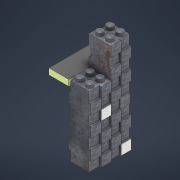
# Autodesk Inventor part: 110033226_ipt_34_中心城堡圍牆
Saved by Autodesk Inventor 2022 (Build 260153000, 153)
## iProperties
Created: 2022-06-24
Part Number: 110033226_ipt_34_中心城堡圍牆
Material: 一般
Document SubType Name: Modeling
Designer: User
Density: 1 g/cm^3
Appearance: 預設
Author: User
Autodesk Inventor part; units mm, degrees
ref_plane "YZ Plane" through (0, 0, 0) normal (1, 0, 0) x (0, 1, 0)
ref_plane "XZ Plane" through (0, 0, 0) normal (0, 1, 0) x (-1, 0, 0)
ref_plane "XY Plane" through (0, 0, 0) normal (0, 0, 1) x (1, 0, 0)
sketch "草圖1" plane through (0, 0, 0) normal (0, 1, 0) x (-1, 0, 0)
  line L0 (2.5, 10) -> (-2.5, 10)
  line L1 (-2.5, 10) -> (-2.5, -10)
  line L2 (-2.5, -10) -> (2.5, -10)
  line L3 (2.5, -10) -> (2.5, 10)
  circle A0 centre (0, 7.5) radius 1.7
  circle A1 centre (0, 2.5) radius 1.7
  circle A2 centre (0, -2.5) radius 1.7
  circle A3 centre (0, -7.5) radius 1.7
  line L4 (2.5, 0) -> (-2.5, 0)
  point P0 (0, 0)
  point P1 (0, -10)
  dimension "d0" = 5
  dimension "d1" = 20
  dimension "d2" = 3.4
  dimension "d3" = 2.5
  dimension "d4" = 2.5
  dimension "d7" = 5
  constraints: 10 end point, 4 centre point, 3 midpoint, 2 parallel, 1 horizontal, 1 horizontal alignment, 1 perpendicular, 1 vertical, 1 vertical alignment, 6 other
  measures "d0" distance of L2.end L1.end
  measures "d1" distance of L1.end L0.end
  measures "d2" diameter of A0
  measures "d3" distance from line of L3 A0.centre
  measures "d4" distance from line of L0 A0.centre
  measures "d7" distance of A0.centre A1.centre
extrude "擠出1" add sketch "草圖1" along normal blind 35 contours L3 L4 L1 L0 | A0 | A1
extrude "擠出2" cut sketch "草圖1" along normal blind 1.5 contours A0 | A1
extrude "擠出3" add sketch "草圖1" along normal blind 50 contours L3 L2 L1 L4 | A2 | A3
extrude "擠出4" cut sketch "草圖1" along normal blind 1.5 contours A2 | A3
sketch "草圖2" plane through (0, 50, 0) normal (0, 1, 0) x (1, 0, 0)
  circle A0 centre (0, 7.5) radius 1.7 projected
  circle A1 centre (0, 2.5) radius 1.7 projected
  point P0 (0, 0)
extrude "擠出5" add sketch "草圖2" along normal blind 1.5
sketch "草圖3" plane through (0, 35, 0) normal (0, 1, 0) x (1, 0, 0)
  circle A0 centre (0, -2.5) radius 1.7 projected
  circle A1 centre (0, -7.5) radius 1.7 projected
  point P0 (0, 0)
extrude "擠出6" add sketch "草圖3" along normal blind 1.5
pattern_linear "矩形陣列1" count 2 spacing 5 along (1, 0, 0) of "擠出6", "擠出5", "擠出4", "擠出3", "擠出2", "擠出1"
sketch "草圖5" plane through (7.5, 0, 10) normal (1, 0, 0) x (0, 0, -1)
  line L0 (0, 0) -> (0, 35) projected
  line L1 (0, 35) -> (10, 35) projected
  line L2 (10, 35) -> (10, 50) projected
  line L3 (10, 50) -> (20, 50) projected
  line L4 (20, 50) -> (20, 0) projected
  line L5 (20, 0) -> (0, 0) projected
  line L6 (20, 0) -> (0, 0) projected
  line L7 (0, 0) -> (20, 0)
  line L8 (0, 5) -> (20, 5)
  line L9 (0, 10) -> (20, 10)
  line L10 (0, 15) -> (20, 15)
  line L11 (0, 20) -> (20, 20)
  line L12 (0, 25) -> (20, 25)
  line L13 (0, 30) -> (20, 30)
  line L14 (0, 35) -> (20, 35)
  line L15 (0, 40) -> (20, 40)
  line L16 (0, 45) -> (20, 45)
  line L17 (20, 0) -> (20, 50) projected
  line L18 (20, 50) -> (20, 0)
  line L19 (15, 50) -> (15, 0)
  line L20 (10, 50) -> (10, 0)
  line L21 (5, 50) -> (5, 0)
  point P0 (5, 5)
  point P1 (5, 10)
  point P2 (5, 15)
  point P3 (5, 20)
  point P4 (5, 25)
  point P5 (5, 30)
  point P6 (10, 5)
  point P7 (10, 10)
  point P8 (10, 15)
  point P9 (10, 20)
  point P10 (10, 25)
  point P11 (5, 35)
  point P12 (10, 30)
  point P13 (15, 5)
  point P14 (15, 10)
  point P15 (15, 15)
  point P16 (15, 20)
  point P17 (15, 25)
  point P18 (15, 30)
  point P19 (15, 35)
  point P20 (15, 40)
  point P21 (10, 40)
  point P22 (15, 45)
  point P23 (10, 45)
  dimension "d29" = 5
  dimension "d39" = 5
  constraints: 28 end point, 2 horizontal, 1 collinear, 1 vertical, 37 other
  measures "d29" distance of L0.start L8.start
  measures "d39" distance of L3.end L19.start
extrude "擠出7" add sketch "草圖5" along normal blind 0.5 contours L0 L9 L21 L8 | L21 L8 L20 L5 | L0 L11 L21 L10 | L21 L10 L20 L9 | L20 L9 L19 L8 | L19 L8 L4 L5 | L0 L13 L21 L12 | L21 L12 L20 L11 | L20 L11 L19 L10 | L19 L10 L4 L9 | L21 L1 L20 L13 | L20 L13 L19 L12 | L2 L15 L19 L14 | L19 L14 L4 L13 | L2 L3 L19 L16 | L19 L16 L4 L15
extrude "擠出8" cut sketch "草圖5" against normal blind 0.5 contours L0 L8 L21 L5 | L0 L10 L21 L9 | L21 L9 L20 L8 | L20 L8 L19 L5 | L0 L12 L21 L11 | L21 L11 L20 L10 | L20 L10 L19 L9 | L19 L9 L4 L8 | L0 L1 L21 L13 | L21 L13 L20 L12 | L20 L12 L19 L11 | L19 L11 L4 L10 | L20 L14 L19 L13 | L19 L13 L4 L12 | L2 L16 L19 L15 | L19 L15 L4 L14 | L19 L3 L4 L16
ref_plane "工作平面1" through (2.5, 0, 10) normal (-1, 0, 0) x (0, 0, 1)
mirror "鏡射1" about plane through (2.5, 0, 10) normal (-1, 0, 0) of "擠出7", "擠出8"
sketch "草圖6" plane through (0, 35, 0) normal (0, 1, 0) x (1, 0, 0)
  line L0 (7, 5) -> (7, 0) projected
  line L1 (8, 0) -> (7, 0) projected
  line L2 (8, 0) -> (8, -5) projected
  line L3 (8, -5) -> (7, -5) projected
  line L4 (7, -5) -> (7, -10) projected
  line L5 (7, -10) -> (-2, -10) projected
  line L6 (-2, -10) -> (-2, -5) projected
  line L7 (-2, -5) -> (-3, -5) projected
  line L8 (-3, -5) -> (-3, 0) projected
  line L9 (-3, 0) -> (-3, 5) projected
  line L10 (-3, 5) -> (-3, 10) projected
  line L11 (-3, 10) -> (-2, 10) projected
  line L12 (-2, 10) -> (7, 10) projected
  line L13 (7, 10) -> (8, 10) projected
  line L14 (8, 10) -> (8, 5) projected
  line L15 (8, 5) -> (8, 0) projected
  line L16 (7, 5) -> (8, 5) projected
  line L17 (7, 10) -> (7, 5) projected
  line L18 (7, 0) -> (-2, 0) projected
  line L19 (-3, 0) -> (-2, 0) projected
  line L20 (-3, 5) -> (-2, 5) projected
  line L21 (-2, 0) -> (-2, 5) projected
  line L22 (-2, 5) -> (-2, 10) projected
  circle A0 centre (5, -2.5) radius 1.7 projected
  circle A1 centre (5, -7.5) radius 1.7 projected
  circle A2 centre (0, -7.5) radius 1.7 projected
  circle A3 centre (0, -2.5) radius 1.7 projected
  line L23 (-3, -5) -> (-3, -10) projected
  line L24 (-3, -10) -> (17, -10)
  line L25 (17, -10) -> (17, 0)
  line L26 (17, 0) -> (-3, 0)
  line L27 (-3, 0) -> (-3, -10)
  line L28 (8, 5) -> (8, 0) projected
  line L29 (8, -5) -> (8, -10) projected
  line L30 (8, 0) -> (8, -10)
  line L31 (-3, 10) -> (8, 10) construction
  line L32 (2.5, 10) -> (2.5, -10) construction
  line L33 (-3, 10) -> (-13, 10)
  line L34 (-13, 10) -> (-13, -10)
  line L35 (-13, -10) -> (-3, -10)
  line L36 (-3, -10) -> (-3, 10) construction
  point P0 (0, 0)
  dimension "d49" = 20
  dimension "d50" = 10
  dimension "d56" = 10
  dimension "d57" = 20
  constraints: 20 end point, 4 parallel, 3 perpendicular, 2 horizontal, 1 collinear, 1 midpoint, 1 point on line
  measures "d49" distance of L26.end L25.end
  measures "d50" distance of L24.end L25.end
  measures "d56" distance of L35.end L34.end
  measures "d57" distance of L34.end L33.end
extrude "擠出10" add sketch "草圖6" against normal blind 3 contours L8 L23 L35 L34 L33 L10 L9
split_face "分割2"
sketch "草圖7" plane through (8, 40, -10) normal (0, 0, -1) x (-1, 0, 0)
  line L0 (1, 5) -> (1, 10) projected
  line L1 (1, 10) -> (10, 10) projected
  line L2 (10, 10) -> (10, 5) projected
  line L3 (10, 5) -> (11, 5) projected
  line L4 (11, 5) -> (11, 0) projected
  line L5 (11, 0) -> (10, 0) projected
  line L6 (10, 0) -> (10, -5) projected
  line L7 (10, -5) -> (11, -5) projected
  line L8 (11, -5) -> (21, -5) projected
  line L9 (21, -5) -> (21, -8) projected
  line L10 (21, -8) -> (11, -8) projected
  line L11 (11, -8) -> (11, -10) projected
  line L12 (11, -10) -> (10, -10) projected
  line L13 (10, -10) -> (10, -15) projected
  line L14 (10, -15) -> (10.5, -15) projected
  line L15 (10.5, -15) -> (10.5, -20) projected
  line L16 (10.5, -20) -> (10, -20) projected
  line L17 (10, -20) -> (10, -25) projected
  line L18 (10, -25) -> (11, -25) projected
  line L19 (11, -25) -> (11, -30) projected
  line L20 (11, -30) -> (10, -30) projected
  line L21 (10, -30) -> (10, -35) projected
  line L22 (10, -35) -> (11, -35) projected
  line L23 (11, -35) -> (11, -40) projected
  line L24 (11, -40) -> (0, -40) projected
  line L25 (0, -40) -> (0, -35) projected
  line L26 (0, -35) -> (1, -35) projected
  line L27 (1, -35) -> (1, -30) projected
  line L28 (1, -30) -> (0, -30) projected
  line L29 (0, -30) -> (0, -25) projected
  line L30 (0, -25) -> (1, -25) projected
  line L31 (1, -25) -> (1, -20) projected
  line L32 (1, -20) -> (0.5, -20) projected
  line L33 (0.5, -20) -> (0.5, -15) projected
  line L34 (0.5, -15) -> (1, -15) projected
  line L35 (1, -15) -> (1, -10) projected
  line L36 (1, -10) -> (0, -10) projected
  line L37 (0, -10) -> (0, -5) projected
  line L38 (0, -5) -> (1, -5) projected
  line L39 (1, -5) -> (1, 0) projected
  line L40 (1, 0) -> (0, 0) projected
  line L41 (0, 0) -> (0, 5) projected
  line L42 (0, 5) -> (1, 5) projected
  line L43 (1, 5) -> (1, 10) projected
  line L44 (1, 10) -> (10, 10) projected
  line L45 (10, 10) -> (10, 5) projected
  line L46 (10, 5) -> (11, 5) projected
  line L47 (11, 5) -> (11, 0) projected
  line L48 (11, 0) -> (10, 0) projected
  line L49 (10, 0) -> (10, -5) projected
  line L50 (10, -5) -> (11, -5) projected
  line L51 (11, -5) -> (21, -5) projected
  line L52 (21, -5) -> (21, -8) projected
  line L53 (21, -8) -> (11, -8) projected
  line L54 (11, -8) -> (11, -10) projected
  line L55 (11, -10) -> (10, -10) projected
  line L56 (10, -10) -> (10, -15) projected
  line L57 (10, -15) -> (10.5, -15) projected
  line L58 (10.5, -15) -> (10.5, -20) projected
  line L59 (10.5, -20) -> (10, -20) projected
  line L60 (10, -20) -> (10, -25) projected
  line L61 (10, -25) -> (11, -25) projected
  line L62 (11, -25) -> (11, -30) projected
  line L63 (11, -30) -> (10, -30) projected
  line L64 (10, -30) -> (10, -35) projected
  line L65 (10, -35) -> (11, -35) projected
  line L66 (11, -35) -> (11, -40) projected
  line L67 (11, -40) -> (0, -40) projected
  line L68 (0, -40) -> (0, -35) projected
  line L69 (0, -35) -> (1, -35) projected
  line L70 (1, -35) -> (1, -30) projected
  line L71 (1, -30) -> (0, -30) projected
  line L72 (0, -30) -> (0, -25) projected
  line L73 (0, -25) -> (1, -25) projected
  line L74 (1, -25) -> (1, -20) projected
  line L75 (1, -20) -> (0.5, -20) projected
  line L76 (0.5, -20) -> (0.5, -15) projected
  line L77 (0.5, -15) -> (1, -15) projected
  line L78 (1, -15) -> (1, -10) projected
  line L79 (1, -10) -> (0, -10) projected
  line L80 (0, -10) -> (0, -5) projected
  line L81 (0, -5) -> (1, -5) projected
  line L82 (1, -5) -> (1, 0) projected
  line L83 (1, 0) -> (0, 0) projected
  line L84 (0, 0) -> (0, 5) projected
  line L85 (0, 5) -> (1, 5) projected
  line L86 (10, -5) -> (11, -5) projected
  line L87 (11, -8) -> (11, -5) projected
  line L88 (11, -5) -> (11, -8)
  point P0 (8, -40)
  constraints: 2 end point, 1 vertical
split_face "分割3"
